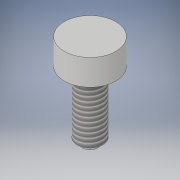
# Autodesk Inventor part: bolt M10x36
Saved by Autodesk Inventor 2018 (Build 220112000, 112)
## iProperties
Created: 2021-03-15
Part Number: bolt M10x36
Material: Generic
Document SubType Name: Modeling
Designer: Jyoti Soni
Density: 1 g/cm^3
Appearance: Default
Mass: 9.09386 g
Surface Area: 30.0426 cm^2
Volume: 9.09386 cm^3
Author: Jyoti Soni
Autodesk Inventor part; units mm, degrees
ref_plane "YZ Plane" through (0, 0, 0) normal (1, 0, 0) x (0, 1, 0)
ref_plane "XZ Plane" through (0, 0, 0) normal (0, 1, 0) x (-1, 0, 0)
ref_plane "XY Plane" through (0, 0, 0) normal (0, 0, 1) x (1, 0, 0)
sketch "Sketch2" plane through (0, 0, 0) normal (0, 0, 1) x (1, 0, 0)
  line L0 (0, 0) -> (0, 36)
  line L1 (0, 36) -> (10, 36)
  line L2 (10, 36) -> (10, 26)
  line L3 (10, 26) -> (5, 26)
  line L4 (5, 26) -> (5, 0)
  line L5 (5, 0) -> (0, 0)
  dimension "d3" = 36
  dimension "d6" = 10
  dimension "d7" = 10
  dimension "d8" = 5
  constraints: 12 end point, 4 perpendicular, 1 horizontal, 1 vertical
  measures "d3" distance of L0.start L0.end
  measures "d6" distance of L0.end L1.end
  measures "d7" distance of L1.end L2.end
  measures "d8" distance of L4.end L0.start
revolve "Revolution1" add sketch "Sketch2" angle 360 about axis through (0, 0, 0) along (0, 1, 0)
chamfer "Chamfer1" distance 2 angle 45 1 edges at (-5, 0, 0)
thread "Thread1" size "M12x1.75" class "6g" standard "ANSI Metric M Profile" full length
body "Solid1"
